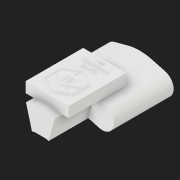
# Autodesk Inventor part: Body
Saved by Autodesk Inventor 2017 SP1 (Build 210196100, 196)
## iProperties
Created: 2018-03-03
Part Number: Body
Material: Generic
Document SubType Name: Modeling
Designer: Zach
Density: 1 g/cm^3
Appearance: CR White
Author: Zach
Autodesk Inventor part; units mm, degrees
ref_plane "YZ Plane" through (0, 0, 0) normal (1, 0, 0) x (0, 1, 0)
ref_plane "XZ Plane" through (0, 0, 0) normal (0, 1, 0) x (-1, 0, 0)
ref_plane "XY Plane" through (0, 0, 0) normal (0, 0, 1) x (1, 0, 0)
sketch "Sketch1" plane through (0, 0, 0) normal (0, 0, 1) x (1, 0, 0)
  line L0 (106.5, -56.5) -> (106.5, 56.5)
  line L1 (38.589, -78.0481) -> (135.1815, -103.93)
  circle A0 centre (155.8871, -26.656) radius 5.25
  line L2 (80, 76.5) -> (176.5926, 50.6181)
  circle A1 centre (155.8871, -26.656) radius 80 construction
  arc A2 (135.1815, -103.93) -> (176.5926, 50.6181) centre (155.8871, -26.656) ccw
  circle A3 centre (-155.8871, -26.656) radius 80 construction
  line L3 (-176.5926, 50.6181) -> (-80, 76.5)
  circle A4 centre (-155.8871, -26.656) radius 5.25
  arc A5 (-176.5926, 50.6181) -> (-135.1815, -103.93) centre (-155.8871, -26.656) ccw
  line L4 (-106.5, 56.5) -> (-106.5, -56.5)
  line L5 (80, 76.5) -> (38.589, -78.0481) construction
  circle A6 centre (0, 71.664) radius 5.25
  line L6 (-38.589, -78.0481) -> (38.589, -78.0481)
  line L7 (-80, 76.5) -> (-38.589, -78.0481) construction
  line L8 (-135.1815, -103.93) -> (-38.589, -78.0481)
  line L9 (-106.5, -56.5) -> (106.5, -56.5)
  line L10 (106.5, 56.5) -> (-106.5, 56.5)
  line L11 (-80, 76.5) -> (80, 76.5) construction
  arc A7 (80, 76.5) -> (-80, 76.5) centre (0, -228.172) ccw
  line L12 (310, 185.5) -> (-310, 185.5) construction
  line L13 (0, 185.5) -> (0, 0) construction
  line L14 (0, 0) -> (310, 0) construction
  line L15 (310, 75.5) -> (310, -324.5) construction
  line L16 (0, -78.0481) -> (0, -56.5)
  point P0 (0, 0)
  point P1 (0, 76.5)
  point P2 (-106.5, 0)
  dimension "d0" = 160
  dimension "d1" = 100
  dimension "d2" = 100
  dimension "d3" = 160
  dimension "d4" = 160
  dimension "d5" = 160
  dimension "d6" = 75
  dimension "d7" = 75
  dimension "d8" = 160
  dimension "d9" = 100
  dimension "d10" = 100
  dimension "d11" = 10.5
  dimension "d12" = 10.5
  dimension "d13" = 113
  dimension "d14" = 213
  dimension "d15" = 20
  dimension "d16" = 315
  dimension "d17" = 10.5
  dimension "d18" = 15.164
  dimension "d19" = 185.5
  constraints: 34 end point, 10 point on circle, 8 centre point, 8 tangent, 5 coincident, 5 midpoint, 3 perpendicular, 2 parallel, 2 point on line, 2 vertical alignment, 1 horizontal alignment, 1 vertical
  measures "d0" diameter of A3
  measures "d1" distance of L11.start L3.start
  measures "d2" distance of L6.start L8.start
  measures "d3" distance of L11.start L6.start
  measures "d4" distance of L11.start L11.end
  measures "d5" distance of L11.end L6.end
  measures "d6" angle of L11 L7
  measures "d7" angle of L11 L5
  measures "d8" diameter of A1
  measures "d9" distance of L6.end L1.end
  measures "d10" distance of L11.end L2.end
  measures "d11" diameter of A4
  measures "d12" diameter of A0
  measures "d13" distance of L10.start L9.end
  measures "d14" distance of L9.end L9.start
  measures "d15" distance between parallel lines of L11 L10
  measures "d16" radius of A7
  measures "d17" diameter of A6
  measures "d18" distance from line of L10 A6.centre
  measures "d19" distance of L13.start L13.end
extrude "Extrusion1" add sketch "Sketch1" along normal blind 70 and the other way blind 345 contours L9 L4 L10 L0 | L6 L8 A5 L3 A7 L2 A2 L1 | A0 | A4 | A6
sketch "Sketch2" plane through (0, 0, 70) normal (0, 0, 1) x (1, 0, 0)
  line L0 (-38.589, -78.0481) -> (38.589, -78.0481) projected
  line L1 (-176.5926, 50.6181) -> (-80, 76.5) projected
  line L2 (-38.589, -78.0481) -> (-80, 76.5)
  line L3 (176.5926, 50.6181) -> (80, 76.5) projected
  line L4 (38.589, -78.0481) -> (80, 76.5)
  arc A0 (80, 76.5) -> (-80, 76.5) centre (0, -228.172) ccw projected
  point P0 (0, 0)
  constraints: 4 end point, 2 perpendicular
extrude "Extrusion2" add sketch "Sketch2" along normal blind 275
ref_plane "Work Plane1" through (-38.589, 76.9519, -345) normal (0, -1, 0) x (1, 0, 0)
sketch "Sketch3" plane through (-38.589, 76.9519, -345) normal (0, -1, 0) x (1, 0, 0)
  line L0 (188.589, 642.5) -> (-111.411, 642.5)
  line L1 (-111.411, 642.5) -> (-111.411, 242.5)
  line L2 (-111.411, 242.5) -> (188.589, 242.5)
  line L3 (188.589, 242.5) -> (188.589, 642.5)
  line L4 (118.589, 690) -> (-41.411, 690) projected
  point P0 (38.589, 345)
  point P1 (38.589, 642.5)
  point P2 (38.589, 690)
  dimension "d25" = 300
  dimension "d26" = 400
  dimension "d27" = 47.5
  constraints: 8 end point, 2 midpoint, 2 parallel, 1 horizontal, 1 perpendicular, 1 vertical alignment
  measures "d25" distance of L2.end L1.end
  measures "d26" distance of L1.end L0.end
  measures "d27" distance between parallel lines of L4 L0
extrude "Extrusion3" add sketch "Sketch3" against normal blind 72
sketch "Sketch4" plane through (-38.589, 148.9519, -345) normal (0, 1, 0) x (1, 0, 0)
  line L0 (188.589, -377.5) -> (-111.411, -377.5) construction
  line L1 (-111.411, -377.5) -> (-111.411, -242.5) construction
  line L2 (-111.411, -242.5) -> (188.589, -242.5) construction
  line L3 (188.589, -242.5) -> (188.589, -377.5) construction
  line L4 (163.589, -627.5) -> (-86.411, -627.5) construction
  line L5 (-86.411, -627.5) -> (-86.411, -377.5) construction
  line L6 (-86.411, -377.5) -> (163.589, -377.5) construction
  line L7 (163.589, -377.5) -> (163.589, -627.5) construction
  line L8 (-111.411, -642.5) -> (188.589, -642.5)
  line L9 (-111.411, -242.5) -> (-111.411, -642.5)
  line L10 (38.589, -627.5) -> (-69.6642, -565)
  line L11 (-69.6642, -565) -> (-69.6642, -440)
  line L12 (-69.6642, -440) -> (38.589, -377.5)
  line L13 (38.589, -377.5) -> (146.8421, -440)
  line L14 (146.8421, -440) -> (146.8421, -565)
  line L15 (146.8421, -565) -> (38.589, -627.5)
  line L16 (38.589, -615.7221) -> (-59.4642, -559.111)
  line L17 (-59.4642, -559.111) -> (-59.4642, -445.889)
  line L18 (-59.4642, -445.889) -> (38.589, -389.2779)
  line L19 (38.589, -389.2779) -> (136.6421, -445.889)
  line L20 (136.6421, -445.889) -> (136.6421, -559.111)
  line L21 (136.6421, -559.111) -> (38.589, -615.7221)
  line L22 (38.589, -610.8146) -> (-55.2142, -556.6573) construction
  line L23 (-55.2142, -556.6573) -> (-55.2142, -448.3427) construction
  line L24 (-55.2142, -448.3427) -> (38.589, -394.1854) construction
  line L25 (38.589, -394.1854) -> (132.3921, -448.3427) construction
  line L26 (132.3921, -448.3427) -> (132.3921, -556.6573) construction
  line L27 (132.3921, -556.6573) -> (38.589, -610.8146) construction
  line L28 (132.3921, -504.1573) -> (92.3921, -527.2513)
  line L29 (92.3921, -527.2513) -> (92.3921, -555.7513)
  line L30 (92.3921, -555.7513) -> (78.3921, -555.7513)
  line L31 (78.3921, -555.7513) -> (78.3921, -535.3342)
  line L32 (78.3921, -535.3342) -> (38.589, -558.3146)
  line L33 (38.589, -558.3146) -> (-55.2142, -504.1573)
  line L34 (-55.2142, -504.1573) -> (-55.2142, -556.6573)
  line L35 (-55.2142, -556.6573) -> (38.589, -610.8146)
  line L36 (38.589, -610.8146) -> (132.3921, -556.6573)
  line L37 (132.3921, -504.1573) -> (132.3921, -556.6573)
  line L38 (132.3921, -448.3427) -> (50.589, -401.1136)
  line L39 (50.589, -401.1136) -> (50.589, -441.1854)
  line L40 (50.589, -441.1854) -> (26.589, -441.1854)
  line L41 (26.589, -441.1854) -> (26.589, -401.1136)
  line L42 (26.589, -401.1136) -> (-55.2142, -448.3427)
  line L43 (-55.2142, -448.3427) -> (-55.2142, -489.1573)
  line L44 (-55.2142, -489.1573) -> (38.589, -543.3146)
  line L45 (38.589, -543.3146) -> (132.3921, -489.1573)
  line L46 (132.3921, -489.1573) -> (132.3921, -448.3427)
  line L47 (64.839, -515.1854) -> (12.339, -515.1854) construction
  line L48 (12.339, -515.1854) -> (12.339, -464.1854) construction
  line L49 (12.339, -464.1854) -> (64.839, -464.1854) construction
  line L50 (64.839, -464.1854) -> (64.839, -515.1854) construction
  line L51 (64.839, -464.1854) -> (40.839, -464.1854)
  line L52 (40.839, -464.1854) -> (40.839, -488.1854)
  line L53 (40.839, -488.1854) -> (64.839, -488.1854)
  line L54 (64.839, -488.1854) -> (64.839, -464.1854)
  line L55 (64.839, -515.1854) -> (40.839, -515.1854)
  line L56 (40.839, -515.1854) -> (40.839, -491.1854)
  line L57 (40.839, -491.1854) -> (64.839, -491.1854)
  line L58 (64.839, -491.1854) -> (64.839, -515.1854)
  line L59 (12.339, -515.1854) -> (36.339, -515.1854)
  line L60 (36.339, -515.1854) -> (36.339, -491.1854)
  line L61 (36.339, -491.1854) -> (12.339, -491.1854)
  line L62 (12.339, -491.1854) -> (12.339, -515.1854)
  line L63 (12.339, -464.1854) -> (36.339, -464.1854)
  line L64 (36.339, -464.1854) -> (36.339, -488.1854)
  line L65 (36.339, -488.1854) -> (12.339, -488.1854)
  line L66 (12.339, -488.1854) -> (12.339, -464.1854)
  line L67 (38.589, -642.5) -> (38.589, -627.5)
  line L68 (38.589, -627.5) -> (38.589, -377.5) construction
  line L69 (188.589, -242.5) -> (-111.411, -242.5) projected
  line L70 (91.8407, -337.3958) -> (91.8407, -341.6804)
  spline S0 degree 2 poles (91.8407, -341.6804) (88.9141, -340.4563) (86.0258, -339.9781) (84.8208, -339.9781) knots 0 0 0 1 2 2 2
  spline S1 degree 2 poles (84.8208, -339.9781) (82.6402, -339.9781) (80.4788, -341.9291) (80.4788, -343.3063) knots 0 0 0 1 2 2 2
  spline S2 degree 2 poles (80.4788, -343.3063) (80.4788, -344.3583) (81.0717, -345.2) knots 0 0 0 1 1 1
  spline S3 degree 2 poles (81.0717, -345.2) (81.6838, -346.0224) (84.0365, -347.3423) knots 0 0 0 1 1 1
  line L71 (84.0365, -347.3423) -> (85.7198, -348.2795)
  spline S4 degree 2 poles (85.7198, -348.2795) (89.3349, -350.2879) (90.5974, -351.9903) knots 0 0 0 1 1 1
  spline S5 degree 2 poles (90.5974, -351.9903) (91.8981, -353.6927) (91.8981, -355.9306) knots 0 0 0 1 1 1
  spline S6 degree 2 poles (91.8981, -355.9306) (91.8981, -358.7615) (87.5752, -362.7784) (83.5392, -362.7784) knots 0 0 0 1 2 2 2
  spline S7 degree 2 poles (83.5392, -362.7784) (80.517, -362.7784) (76.7297, -361.9176) knots 0 0 0 1 1 1
  line L72 (76.7297, -361.9176) -> (76.7297, -357.9199)
  spline S8 degree 2 poles (76.7297, -357.9199) (80.6127, -359.3545) (82.8889, -359.3545) knots 0 0 0 1 1 1
  spline S9 degree 2 poles (82.8889, -359.3545) (84.7825, -359.3545) (86.7527, -357.7095) (86.7527, -356.5618) knots 0 0 0 1 2 2 2
  spline S10 degree 2 poles (86.7527, -356.5618) (86.7527, -355.682) (86.1406, -354.936) knots 0 0 0 1 1 1
  spline S11 degree 2 poles (86.1406, -354.936) (85.5668, -354.1709) (83.214, -352.8511) knots 0 0 0 1 1 1
  line L73 (83.214, -352.8511) -> (81.416, -351.8564)
  spline S12 degree 2 poles (81.416, -351.8564) (77.2653, -349.542) (76.1368, -347.8396) knots 0 0 0 1 1 1
  spline S13 degree 2 poles (76.1368, -347.8396) (75.0082, -346.1181) (75.0082, -343.9758) knots 0 0 0 1 1 1
  spline S14 degree 2 poles (75.0082, -343.9758) (75.0082, -340.8962) (79.6945, -336.5542) (84.8017, -336.5542) knots 0 0 0 1 2 2 2
  spline S15 degree 2 poles (84.8017, -336.5542) (87.8238, -336.5542) (91.8407, -337.3958) knots 0 0 0 1 1 1
  line L74 (70.6854, -337.1663) -> (70.6854, -362.1663)
  line L75 (70.6854, -362.1663) -> (65.4826, -362.1663)
  line L76 (65.4826, -362.1663) -> (65.4826, -340.7049)
  line L77 (65.4826, -340.7049) -> (54.3311, -340.7049)
  line L78 (54.3311, -340.7049) -> (54.3311, -337.1663)
  line L79 (54.3311, -337.1663) -> (70.6854, -337.1663)
  line L80 (53.3173, -337.1663) -> (43.6196, -362.1663)
  line L81 (43.6196, -362.1663) -> (38.3977, -362.1663)
  line L82 (38.3977, -362.1663) -> (28.6616, -337.1663)
  line L83 (28.6616, -337.1663) -> (33.9983, -337.1663)
  line L84 (33.9983, -337.1663) -> (36.5997, -343.8419)
  line L85 (36.5997, -343.8419) -> (46.9287, -343.8419)
  line L86 (46.9287, -343.8419) -> (49.53, -337.1663)
  line L87 (49.53, -337.1663) -> (53.3173, -337.1663)
  line L88 (45.6471, -347.1701) -> (37.9004, -347.1701)
  line L89 (37.9004, -347.1701) -> (41.7642, -357.1357)
  line L90 (41.7642, -357.1357) -> (45.6471, -347.1701)
  line L91 (18.9065, -337.1663) -> (18.9065, -358.7233)
  line L92 (18.9065, -358.7233) -> (27.8583, -358.7233)
  line L93 (27.8583, -358.7233) -> (27.8583, -362.1663)
  line L94 (27.8583, -362.1663) -> (4.7519, -362.1663)
  line L95 (4.7519, -362.1663) -> (4.7519, -358.7233)
  line L96 (4.7519, -358.7233) -> (13.7037, -358.7233)
  line L97 (13.7037, -358.7233) -> (13.7037, -337.1663)
  line L98 (13.7037, -337.1663) -> (18.9065, -337.1663)
  line L99 (1.2707, -337.1663) -> (1.2707, -362.1663)
  line L100 (1.2707, -362.1663) -> (-14.7393, -362.1663)
  line L101 (-14.7393, -362.1663) -> (-14.7393, -358.7233)
  line L102 (-14.7393, -358.7233) -> (-3.9321, -358.7233)
  line L103 (-3.9321, -358.7233) -> (-3.9321, -351.7608)
  line L104 (-3.9321, -351.7608) -> (-12.8648, -351.7608)
  line L105 (-12.8648, -351.7608) -> (-12.8648, -348.3178)
  line L106 (-12.8648, -348.3178) -> (-3.9321, -348.3178)
  line L107 (-3.9321, -348.3178) -> (-3.9321, -340.7049)
  line L108 (-3.9321, -340.7049) -> (-15.5426, -340.7049)
  line L109 (-15.5426, -340.7049) -> (-15.5426, -337.1663)
  line L110 (-15.5426, -337.1663) -> (1.2707, -337.1663)
  line L111 (126.6054, -297.2098) -> (126.6054, -322.2098)
  line L112 (126.6054, -322.2098) -> (117.2519, -322.2098)
  spline S16 degree 2 poles (117.2519, -322.2098) (114.3828, -322.2098) (111.3797, -320.7752) (109.6391, -317.8486) (109.6391, -316.0124) knots 0 0 0 1 2 3 3 3
  spline S17 degree 2 poles (109.6391, -316.0124) (109.6391, -313.8127) (112.1639, -309.9106) (114.4784, -308.8777) knots 0 0 0 1 2 2 2
  line L113 (114.4784, -308.8777) -> (106.3108, -297.2098)
  line L114 (106.3108, -297.2098) -> (112.6421, -297.2098)
  line L115 (112.6421, -297.2098) -> (118.8586, -307.424)
  line L116 (118.8586, -307.424) -> (121.7087, -307.424)
  line L117 (121.7087, -307.424) -> (121.7087, -297.2098)
  line L118 (121.7087, -297.2098) -> (126.6054, -297.2098)
  line L119 (121.7087, -310.8479) -> (120.5228, -310.8479)
  spline S18 degree 2 poles (120.5228, -310.8479) (117.3093, -310.8479) (114.8418, -313.6597) (114.8418, -315.4385) knots 0 0 0 1 2 2 2
  spline S19 degree 2 poles (114.8418, -315.4385) (114.8418, -316.9688) (116.8311, -318.7859) (119.8915, -318.7859) knots 0 0 0 1 2 2 2
  line L120 (119.8915, -318.7859) -> (121.7087, -318.7859)
  line L121 (121.7087, -318.7859) -> (121.7087, -310.8479)
  spline S20 degree 2 poles (91.6207, -296.5977) (95.5228, -296.5977) (101.2994, -299.8303) (104.3024, -305.8747) (104.3024, -309.7193) knots 0 0 0 1 2 3 3 3
  spline S21 degree 2 poles (104.3024, -309.7193) (104.3024, -313.5258) (101.2994, -319.6084) (95.4845, -322.8219) (91.6207, -322.8219) knots 0 0 0 1 2 3 3 3
  spline S22 degree 2 poles (91.6207, -322.8219) (87.776, -322.8219) (81.9612, -319.6084) (78.9581, -313.5258) (78.9581, -309.7193) knots 0 0 0 1 2 3 3 3
  spline S23 degree 2 poles (78.9581, -309.7193) (78.9581, -305.8747) (81.9612, -299.8303) (87.7186, -296.5977) (91.6207, -296.5977) knots 0 0 0 1 2 3 3 3
  spline S24 degree 2 poles (91.6207, -300.0216) (88.0056, -300.0216) (84.486, -305.9129) (84.486, -309.7193) knots 0 0 0 1 2 2 2
  spline S25 degree 2 poles (84.486, -309.7193) (84.486, -313.5449) (88.0247, -319.398) (91.6207, -319.398) knots 0 0 0 1 2 2 2
  spline S26 degree 2 poles (91.6207, -319.398) (95.2358, -319.398) (98.7745, -313.5449) (98.7745, -309.7193) knots 0 0 0 1 2 2 2
  spline S27 degree 2 poles (98.7745, -309.7193) (98.7745, -305.9129) (95.255, -300.0216) (91.6207, -300.0216) knots 0 0 0 1 2 2 2
  line L122 (74.2909, -297.2098) -> (74.2909, -322.2098)
  line L123 (74.2909, -322.2098) -> (65.8556, -322.2098)
  spline S28 degree 2 poles (65.8556, -322.2098) (62.7951, -322.2098) (59.8686, -320.8326) (58.2045, -318.1547) (58.2045, -316.6436) knots 0 0 0 1 2 3 3 3
  spline S29 degree 2 poles (58.2045, -316.6436) (58.2045, -314.7691) (60.8059, -311.3261) (64.1723, -310.274) knots 0 0 0 1 2 2 2
  spline S30 degree 2 poles (64.1723, -310.274) (61.4945, -309.6046) (58.6635, -307.6535) (57.1907, -304.9374) (57.1907, -303.388) knots 0 0 0 1 2 3 3 3
  spline S31 degree 2 poles (57.1907, -303.388) (57.1907, -301.7048) (58.9122, -298.7783) (61.9344, -297.2098) (65.0713, -297.2098) knots 0 0 0 1 2 3 3 3
  line L124 (65.0713, -297.2098) -> (74.2909, -297.2098)
  line L125 (69.2986, -300.7484) -> (68.3039, -300.7484)
  spline S32 degree 2 poles (68.3039, -300.7484) (65.5878, -300.7484) (63.6176, -301.4561) (62.623, -303.0437) (62.623, -304.0193) knots 0 0 0 1 2 3 3 3
  spline S33 degree 2 poles (62.623, -304.0193) (62.623, -305.8747) (65.8938, -308.4569) (68.3996, -308.4569) knots 0 0 0 1 2 2 2
  line L126 (68.3996, -308.4569) -> (69.2986, -308.4569)
  line L127 (69.2986, -308.4569) -> (69.2986, -300.7484)
  line L128 (69.2986, -311.8043) -> (68.1892, -311.8043)
  spline S34 degree 2 poles (68.1892, -311.8043) (65.8173, -311.8043) (63.4837, -314.157) (63.4837, -315.8402) knots 0 0 0 1 2 2 2
  spline S35 degree 2 poles (63.4837, -315.8402) (63.4837, -316.7392) (64.1723, -318.0591) (65.913, -318.7859) (68.3613, -318.7859) knots 0 0 0 1 2 3 3 3
  line L129 (68.3613, -318.7859) -> (69.2986, -318.7859)
  line L130 (69.2986, -318.7859) -> (69.2986, -311.8043)
  spline S36 degree 2 poles (41.372, -296.5977) (45.2741, -296.5977) (51.0507, -299.8303) (54.0538, -305.8747) (54.0538, -309.7193) knots 0 0 0 1 2 3 3 3
  spline S37 degree 2 poles (54.0538, -309.7193) (54.0538, -313.5258) (51.0507, -319.6084) (45.2358, -322.8219) (41.372, -322.8219) knots 0 0 0 1 2 3 3 3
  spline S38 degree 2 poles (41.372, -322.8219) (37.5274, -322.8219) (31.7125, -319.6084) (28.7095, -313.5258) (28.7095, -309.7193) knots 0 0 0 1 2 3 3 3
  spline S39 degree 2 poles (28.7095, -309.7193) (28.7095, -305.8747) (31.7125, -299.8303) (37.47, -296.5977) (41.372, -296.5977) knots 0 0 0 1 2 3 3 3
  spline S40 degree 2 poles (41.372, -300.0216) (37.7569, -300.0216) (34.2374, -305.9129) (34.2374, -309.7193) knots 0 0 0 1 2 2 2
  spline S41 degree 2 poles (34.2374, -309.7193) (34.2374, -313.5449) (37.776, -319.398) (41.372, -319.398) knots 0 0 0 1 2 2 2
  spline S42 degree 2 poles (41.372, -319.398) (44.9872, -319.398) (48.5258, -313.5449) (48.5258, -309.7193) knots 0 0 0 1 2 2 2
  spline S43 degree 2 poles (48.5258, -309.7193) (48.5258, -305.9129) (45.0063, -300.0216) (41.372, -300.0216) knots 0 0 0 1 2 2 2
  line L131 (17.8257, -297.2098) -> (17.8257, -318.7668)
  line L132 (17.8257, -318.7668) -> (26.7775, -318.7668)
  line L133 (26.7775, -318.7668) -> (26.7775, -322.2098)
  line L134 (26.7775, -322.2098) -> (3.6712, -322.2098)
  line L135 (3.6712, -322.2098) -> (3.6712, -318.7668)
  line L136 (3.6712, -318.7668) -> (12.623, -318.7668)
  line L137 (12.623, -318.7668) -> (12.623, -297.2098)
  line L138 (12.623, -297.2098) -> (17.8257, -297.2098)
  line L139 (0.1899, -297.2098) -> (0.1899, -322.2098)
  line L140 (0.1899, -322.2098) -> (-5.0128, -322.2098)
  line L141 (-5.0128, -322.2098) -> (-5.0128, -297.2098)
  line L142 (-5.0128, -297.2098) -> (0.1899, -297.2098)
  spline S44 degree 2 poles (-31.39, -298.2044) (-29.745, -297.4776) (-27.3158, -296.942) (-24.2362, -296.5977) (-22.7251, -296.5977) knots 0 0 0 1 2 3 3 3
  spline S45 degree 2 poles (-22.7251, -296.5977) (-16.1643, -296.5977) (-9.7182, -303.981) (-9.7182, -309.7193) knots 0 0 0 1 2 2 2
  spline S46 degree 2 poles (-9.7182, -309.7193) (-9.7182, -315.4577) (-16.1452, -322.8219) (-23.0503, -322.8219) knots 0 0 0 1 2 2 2
  spline S47 degree 2 poles (-23.0503, -322.8219) (-27.1245, -322.8219) (-31.1605, -321.8655) knots 0 0 0 1 1 1
  line L143 (-31.1605, -321.8655) -> (-31.1605, -317.7913)
  spline S48 degree 2 poles (-31.1605, -317.7913) (-29.2094, -318.4607) (-26.742, -319.092) (-24.5423, -319.398) (-23.4329, -319.398) knots 0 0 0 1 2 3 3 3
  spline S49 degree 2 poles (-23.4329, -319.398) (-19.1291, -319.398) (-15.2462, -313.8701) (-15.2462, -309.7767) knots 0 0 0 1 2 2 2
  spline S50 degree 2 poles (-15.2462, -309.7767) (-15.2462, -305.4921) (-19.6456, -300.1937) (-24.0067, -300.1937) knots 0 0 0 1 2 2 2
  spline S51 degree 2 poles (-24.0067, -300.1937) (-27.641, -300.1937) (-31.39, -302.03) knots 0 0 0 1 1 1
  line L144 (-31.39, -302.03) -> (-31.39, -298.2044)
  line L145 (-34.5078, -297.4393) -> (-34.5078, -301.7239)
  spline S52 degree 2 poles (-34.5078, -301.7239) (-37.4344, -300.4998) (-40.3227, -300.0216) (-41.5277, -300.0216) knots 0 0 0 1 2 2 2
  spline S53 degree 2 poles (-41.5277, -300.0216) (-43.7083, -300.0216) (-45.8697, -301.9726) (-45.8697, -303.3498) knots 0 0 0 1 2 2 2
  spline S54 degree 2 poles (-45.8697, -303.3498) (-45.8697, -304.4018) (-45.2768, -305.2434) knots 0 0 0 1 1 1
  spline S55 degree 2 poles (-45.2768, -305.2434) (-44.6647, -306.0659) (-42.312, -307.3858) knots 0 0 0 1 1 1
  line L146 (-42.312, -307.3858) -> (-40.6287, -308.323)
  spline S56 degree 2 poles (-40.6287, -308.323) (-37.0136, -310.3314) (-35.7511, -312.0338) knots 0 0 0 1 1 1
  spline S57 degree 2 poles (-35.7511, -312.0338) (-34.4505, -313.7362) (-34.4505, -315.9741) knots 0 0 0 1 1 1
  spline S58 degree 2 poles (-34.4505, -315.9741) (-34.4505, -318.805) (-38.7733, -322.8219) (-42.8093, -322.8219) knots 0 0 0 1 2 2 2
  spline S59 degree 2 poles (-42.8093, -322.8219) (-45.8315, -322.8219) (-49.6188, -321.9611) knots 0 0 0 1 1 1
  line L147 (-49.6188, -321.9611) -> (-49.6188, -317.9634)
  spline S60 degree 2 poles (-49.6188, -317.9634) (-45.7358, -319.398) (-43.4596, -319.398) knots 0 0 0 1 1 1
  spline S61 degree 2 poles (-43.4596, -319.398) (-41.566, -319.398) (-39.5958, -317.753) (-39.5958, -316.6053) knots 0 0 0 1 2 2 2
  spline S62 degree 2 poles (-39.5958, -316.6053) (-39.5958, -315.7255) (-40.2079, -314.9795) knots 0 0 0 1 1 1
  spline S63 degree 2 poles (-40.2079, -314.9795) (-40.7817, -314.2144) (-43.1345, -312.8946) knots 0 0 0 1 1 1
  line L148 (-43.1345, -312.8946) -> (-44.9325, -311.8999)
  spline S64 degree 2 poles (-44.9325, -311.8999) (-49.0832, -309.5854) (-50.2117, -307.8831) knots 0 0 0 1 1 1
  spline S65 degree 2 poles (-50.2117, -307.8831) (-51.3403, -306.1616) (-51.3403, -304.0193) knots 0 0 0 1 1 1
  spline S66 degree 2 poles (-51.3403, -304.0193) (-51.3403, -300.9397) (-46.654, -296.5977) (-41.5469, -296.5977) knots 0 0 0 1 2 2 2
  spline S67 degree 2 poles (-41.5469, -296.5977) (-38.5247, -296.5977) (-34.5078, -297.4393) knots 0 0 0 1 1 1
  line L149 (62.2428, -257.2216) -> (57.7813, -279.5678)
  line L150 (57.7813, -279.5678) -> (66.6659, -279.5678)
  line L151 (66.6659, -279.5678) -> (66.1466, -282.2216)
  line L152 (66.1466, -282.2216) -> (44.8582, -282.2216)
  line L153 (44.8582, -282.2216) -> (45.3966, -279.5678)
  line L154 (45.3966, -279.5678) -> (54.262, -279.5678)
  line L155 (54.262, -279.5678) -> (58.7043, -257.2216)
  line L156 (58.7043, -257.2216) -> (62.2428, -257.2216)
  line L157 (46.4543, -257.2216) -> (41.4736, -282.2216)
  line L158 (41.4736, -282.2216) -> (33.9351, -282.2216)
  spline S68 degree 2 poles (33.9351, -282.2216) (31.9543, -282.2216) (29.2428, -281.5485) (27.4543, -279.1255) (27.4543, -277.3755) knots 0 0 0 1 2 3 3 3
  spline S69 degree 2 poles (27.4543, -277.3755) (27.4543, -274.837) (31.0697, -270.337) (34.1466, -269.1639) knots 0 0 0 1 2 2 2
  line L159 (34.1466, -269.1639) -> (28.2043, -257.2216)
  line L160 (28.2043, -257.2216) -> (32.1274, -257.2216)
  line L161 (32.1274, -257.2216) -> (37.3774, -268.2793)
  line L162 (37.3774, -268.2793) -> (40.7236, -268.2793)
  line L163 (40.7236, -268.2793) -> (42.9159, -257.2216)
  line L164 (42.9159, -257.2216) -> (46.4543, -257.2216)
  line L165 (40.2043, -270.8947) -> (38.2428, -270.8947)
  spline S70 degree 2 poles (38.2428, -270.8947) (36.1466, -270.8947) (33.0505, -272.4716) (31.2236, -275.4716) (31.2236, -276.9716) knots 0 0 0 1 2 3 3 3
  spline S71 degree 2 poles (31.2236, -276.9716) (31.2236, -278.2601) (33.1851, -279.5678) (36.2236, -279.5678) knots 0 0 0 1 2 2 2
  line L166 (36.2236, -279.5678) -> (38.4736, -279.5678)
  line L167 (38.4736, -279.5678) -> (40.2043, -270.8947)
  line L168 (18.762, -257.2216) -> (14.2813, -279.6832)
  line L169 (14.2813, -279.6832) -> (18.1851, -279.6832)
  line L170 (18.1851, -279.6832) -> (17.762, -281.7601)
  line L171 (17.762, -281.7601) -> (10.3774, -282.4332)
  line L172 (10.3774, -282.4332) -> (15.4351, -257.2216)
  line L173 (15.4351, -257.2216) -> (18.762, -257.2216)
  point P0 (38.589, -345)
  point P1 (38.589, -502.5)
  point P2 (38.589, -441.1854)
  point P3 (38.589, -515.1854)
  point P4 (38.589, -464.1854)
  point P5 (38.589, -242.5)
  dimension "d30" = 15
  dimension "d31" = 250
  dimension "d32" = 10.2
  dimension "d33" = 4.25
  dimension "d34" = 52.5
  dimension "d35" = 40
  dimension "d36" = 14
  dimension "d37" = 28.5
  dimension "d38" = 15
  dimension "d39" = 24
  dimension "d40" = 47
  dimension "d41" = 23
  dimension "d42" = 51
  dimension "d43" = 52.5
  dimension "d44" = 24
  dimension "d45" = 24
  dimension "d46" = 24
  dimension "d47" = 24
  dimension "d48" = 24
  dimension "d49" = 24
  dimension "d50" = 24
  dimension "d51" = 24
  dimension "d54" = 300
  dimension "d56" = 400
  constraints: 122 end point, 16 parallel, 16 perpendicular, 12 point on line, 9 midpoint, 4 collinear, 1 coincident, 1 horizontal, 26 other
  measures "d30" distance between parallel lines of L8 L4
  measures "d31" distance of L7.end L5.start
  measures "d32" distance between parallel lines of L15 L21
  measures "d33" distance between parallel lines of L21 L27
  measures "d34" distance of L28.start L37.end
  measures "d35" distance between parallel lines of L26 L29
  measures "d36" distance of L30.start L30.end
  measures "d37" distance of L29.start L30.start
  measures "d38" distance of L33.start L44.end
  measures "d39" distance between parallel lines of L41 L39
  measures "d40" distance from line of L24.end L40
  measures "d41" distance between parallel lines of L40 L49
  measures "d42" distance of L51.start L55.start
  measures "d43" distance of L55.start L62.end
  measures "d44" distance of L53.end L53.start
  measures "d45" distance of L53.start L51.end
  measures "d46" distance of L56.end L57.end
  measures "d47" distance of L55.end L56.end
  measures "d48" distance of L61.end L61.start
  measures "d49" distance of L61.start L60.start
  measures "d50" distance of L64.end L66.start
  measures "d51" distance of L64.start L64.end
  measures "d54" distance of L9.end L8.end
  measures "d56" distance of L9.start L9.end
extrude "Extrusion4" add sketch "Sketch4" along normal blind 2
sketch "Sketch5" plane through (0, 0, 70) normal (0, 0, 1) x (1, 0, 0)
  line L0 (-80, 76.5) -> (-38.589, -78.0481) projected
  line L1 (38.589, -78.0481) -> (80, 76.5) projected
  line L2 (-80, 76.5) -> (-99.3185, 71.3236)
  line L3 (-176.5926, 50.6181) -> (-80, 76.5) projected
  line L4 (-99.3185, 71.3236) -> (-57.9075, -83.2245)
  line L5 (-38.589, -78.0481) -> (-135.1815, -103.93) projected
  line L6 (38.589, -78.0481) -> (-38.589, -78.0481) projected
  line L7 (-38.589, -78.0481) -> (-57.9075, -83.2245)
  line L8 (80, 76.5) -> (38.589, -78.0481)
  line L9 (57.9075, -83.2245) -> (99.3185, 71.3236)
  line L10 (99.3185, 71.3236) -> (80, 76.5)
  line L11 (135.1815, -103.93) -> (38.589, -78.0481) projected
  line L12 (57.9075, -83.2245) -> (38.589, -78.0481)
  point P0 (0, 0)
  dimension "d98" = 20
  dimension "d99" = 20
  constraints: 14 end point, 2 collinear, 2 perpendicular, 2 point on line, 1 parallel
  measures "d98" distance of L0.start L2.end
  measures "d99" distance of L9.start L1.start
extrude "Extrusion5" add sketch "Sketch5" along normal blind 275
body "Solid1"
